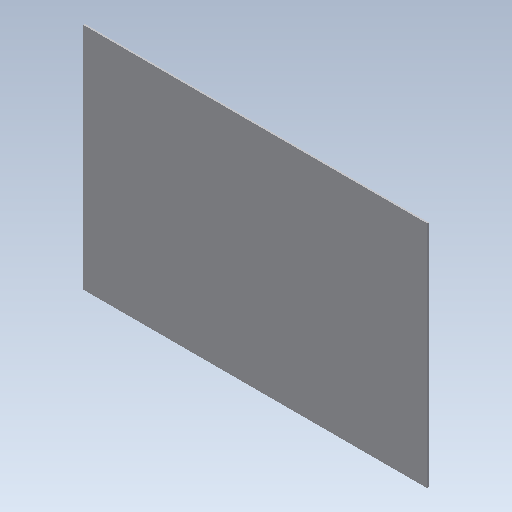
# Autodesk Inventor part: solar1
Saved by Autodesk Inventor 2020 (Build 240168000, 168)
## iProperties
Created: 2016-11-10
Part Number: solar1
Material: Aluminum 6061-AHC
Document SubType Name: Modeling
Designer: jous
Density: 2.71 g/cm^3
Appearance: Aluminum - Dark
Mass: 612.494 g
Surface Area: 2382.82 cm^2
Volume: 226.012 cm^3
Author: jous
Autodesk Inventor part; units mm, degrees
ref_plane "YZ Plane" through (0, 0, 0) normal (1, 0, 0) x (0, 1, 0)
ref_plane "XZ Plane" through (0, 0, 0) normal (0, 1, 0) x (-1, 0, 0)
ref_plane "XY Plane" through (0, 0, 0) normal (0, 0, 1) x (1, 0, 0)
sketch "Sketch1" plane through (0, 0, 0) normal (0, 0, 1) x (1, 0, 0)
  line L0 (-300, -140) -> (120, -140)
  line L1 (120, -140) -> (120, 140)
  line L2 (120, 140) -> (-300, 140)
  line L3 (-300, 140) -> (-300, -140)
  point P0 (0, 0)
  dimension "d0" = 420
  dimension "d1" = 280
  dimension "d36" = 300
  constraints: 8 end point, 2 parallel, 1 horizontal, 1 perpendicular
  measures "d0" distance of L2.end L1.end
  measures "d1" distance of L1.end L0.end
  measures "d36" distance from line of point (0, 0) L3
sketch "Sketch4" plane through (0, 0, 0) normal (0, 0, 1) x (1, 0, 0)
  line L0 (-273, -1) -> (-260.5, -1)
  line L1 (-148, -1) -> (-148, -13.5)
  line L2 (-148, -126) -> (-160.5, -126)
  line L3 (-273, -126) -> (-273, -113.5)
  line L4 (-273, -13.5) -> (-260.5, -1)
  line L5 (-160.5, -1) -> (-148, -13.5)
  line L6 (-148, -113.5) -> (-160.5, -126)
  line L7 (-260.5, -126) -> (-273, -113.5)
  line L8 (-260.5, -1) -> (-160.5, -1)
  line L9 (-273, -13.5) -> (-273, -1)
  line L10 (-160.5, -1) -> (-148, -1)
  line L11 (-148, -13.5) -> (-148, -113.5)
  line L12 (-160.5, -126) -> (-260.5, -126)
  line L13 (-148, -113.5) -> (-148, -126)
  line L14 (-260.5, -126) -> (-273, -126)
  line L15 (-273, -113.5) -> (-273, -13.5)
  line L16 (-300, -140) -> (120, -140) projected
  line L17 (-300, 140) -> (-300, -140) projected
  point P0 (0, 0)
  dimension "d6" = 125
  dimension "d7" = 125
  dimension "d8" = 12.5
  dimension "d9" = 12.5
  dimension "d10" = 12.5
  dimension "d11" = 12.5
  dimension "d12" = 12.5
  dimension "d13" = 12.5
  dimension "d14" = 12.5
  dimension "d15" = 12.5
  dimension "d22" = 14
  dimension "d23" = 27
  constraints: 32 end point, 18 parallel, 9 perpendicular, 3 horizontal, 3 point on line
  measures "d6" distance of L2.start L3.start
  measures "d7" distance of L1.start L2.start
  measures "d8" distance of L0.end L0.start
  measures "d9" distance of L1.start L5.start
  measures "d10" distance of L1.end L1.start
  measures "d11" distance of L2.start L6.start
  measures "d12" distance of L2.end L2.start
  measures "d13" distance of L3.start L7.start
  measures "d14" distance of L3.end L3.start
  measures "d15" distance of L4.start L0.start
  measures "d22" distance between parallel lines of L12 L16
  measures "d23" distance between parallel lines of L15 L17
sketch "Sketch5" plane through (0, 0, 0) normal (0, 0, 1) x (1, 0, 0)
  line L0 (-273, -13.5) -> (-260.5, -1) projected
  line L1 (-260.5, -1) -> (-160.5, -1) projected
  line L2 (-160.5, -1) -> (-148, -13.5) projected
  line L3 (-148, -13.5) -> (-148, -113.5) projected
  line L4 (-160.5, -126) -> (-260.5, -126) projected
  line L5 (-148, -113.5) -> (-160.5, -126) projected
  line L6 (-260.5, -126) -> (-273, -113.5) projected
  line L7 (-273, -113.5) -> (-273, -13.5) projected
  point P0 (0, 0)
boundary_patch "Boundary Patch3"
pattern_linear "Rectangular Pattern1" count 3 spacing 127 along (1, 0, 0) count 2 spacing 127 along (0, 1, 0) of "Boundary Patch3"
sketch "Sketch6" plane through (0, 0, 0) normal (0, 0, 1) x (1, 0, 0)
  line L0 (120, 140) -> (-300, 140) projected
  line L1 (-300, 140) -> (-300, -140) projected
  line L2 (-300, -140) -> (120, -140) projected
  line L3 (120, -140) -> (120, 140) projected
  line L4 (-260.5, 126) -> (-160.5, 126) projected
  line L5 (-133.5, 126) -> (-33.5, 126) projected
  line L6 (-146, 113.5) -> (-133.5, 126) projected
  line L7 (-160.5, 126) -> (-148, 113.5) projected
  line L8 (-273, 13.5) -> (-273, 113.5) projected
  line L9 (-273, 113.5) -> (-260.5, 126) projected
  line L10 (-260.5, 1) -> (-273, 13.5) projected
  line L11 (-160.5, 1) -> (-260.5, 1) projected
  line L12 (-148, 113.5) -> (-148, 13.5) projected
  line L13 (-148, 13.5) -> (-160.5, 1) projected
  line L14 (-133.5, 1) -> (-146, 13.5) projected
  line L15 (-146, 13.5) -> (-146, 113.5) projected
  line L16 (-21, 113.5) -> (-21, 13.5) projected
  line L17 (-19, 13.5) -> (-19, 113.5) projected
  line L18 (-33.5, 126) -> (-21, 113.5) projected
  line L19 (-19, 113.5) -> (-6.5, 126) projected
  line L20 (-6.5, 126) -> (93.5, 126) projected
  line L21 (93.5, 126) -> (106, 113.5) projected
  line L22 (106, 113.5) -> (106, 13.5) projected
  line L23 (-273, -113.5) -> (-273, -13.5) projected
  line L24 (-273, -13.5) -> (-260.5, -1) projected
  line L25 (-160.5, -1) -> (-148, -13.5) projected
  line L26 (-260.5, -1) -> (-160.5, -1) projected
  line L27 (-146, -13.5) -> (-133.5, -1) projected
  line L28 (-33.5, -1) -> (-21, -13.5) projected
  line L29 (-133.5, -1) -> (-33.5, -1) projected
  line L30 (-33.5, 1) -> (-133.5, 1) projected
  line L31 (-21, 13.5) -> (-33.5, 1) projected
  line L32 (106, 13.5) -> (93.5, 1) projected
  line L33 (-6.5, 1) -> (-19, 13.5) projected
  line L34 (93.5, 1) -> (-6.5, 1) projected
  line L35 (-6.5, -1) -> (93.5, -1) projected
  line L36 (-19, -13.5) -> (-6.5, -1) projected
  line L37 (93.5, -1) -> (106, -13.5) projected
  line L38 (-160.5, -126) -> (-260.5, -126) projected
  line L39 (-148, -13.5) -> (-148, -113.5) projected
  line L40 (-146, -113.5) -> (-146, -13.5) projected
  line L41 (-21, -13.5) -> (-21, -113.5) projected
  line L42 (-19, -113.5) -> (-19, -13.5) projected
  line L43 (106, -13.5) -> (106, -113.5) projected
  line L44 (106, -113.5) -> (93.5, -126) projected
  line L45 (93.5, -126) -> (-6.5, -126) projected
  line L46 (-6.5, -126) -> (-19, -113.5) projected
  line L47 (-21, -113.5) -> (-33.5, -126) projected
  line L48 (-33.5, -126) -> (-133.5, -126) projected
  line L49 (-133.5, -126) -> (-146, -113.5) projected
  line L50 (-148, -113.5) -> (-160.5, -126) projected
  line L51 (-260.5, -126) -> (-273, -113.5) projected
  point P0 (0, 0)
sketch "Sketch9" plane through (0, 0, 0) normal (0, 0, 1) x (1, 0, 0)
  line L0 (-260.5, 126) -> (-160.5, 126) projected
  line L1 (-160.5, 126) -> (-148, 113.5) projected
  line L2 (-148, 113.5) -> (-148, 13.5) projected
  line L3 (-273, 13.5) -> (-273, 113.5) projected
  line L4 (-273, 113.5) -> (-260.5, 126) projected
  line L5 (-160.5, 1) -> (-260.5, 1) projected
  line L6 (-260.5, 1) -> (-273, 13.5) projected
  line L7 (-273, -13.5) -> (-260.5, -1) projected
  line L8 (-260.5, -1) -> (-160.5, -1) projected
  line L9 (-273, -113.5) -> (-273, -13.5) projected
  line L10 (-160.5, -1) -> (-148, -13.5) projected
  line L11 (-148, -13.5) -> (-148, -113.5) projected
  line L12 (-148, 13.5) -> (-160.5, 1) projected
  line L13 (-133.5, 1) -> (-146, 13.5) projected
  line L14 (-146, -13.5) -> (-133.5, -1) projected
  line L15 (-146, -113.5) -> (-146, -13.5) projected
  line L16 (-146, 13.5) -> (-146, 113.5) projected
  line L17 (-133.5, 126) -> (-33.5, 126) projected
  line L18 (-146, 113.5) -> (-133.5, 126) projected
  line L19 (-33.5, 126) -> (-21, 113.5) projected
  line L20 (-21, 113.5) -> (-21, 13.5) projected
  line L21 (-21, 13.5) -> (-33.5, 1) projected
  line L22 (-33.5, 1) -> (-133.5, 1) projected
  line L23 (-133.5, -1) -> (-33.5, -1) projected
  line L24 (-33.5, -126) -> (-133.5, -126) projected
  line L25 (-160.5, -126) -> (-260.5, -126) projected
  line L26 (-260.5, -126) -> (-273, -113.5) projected
  line L27 (-148, -113.5) -> (-160.5, -126) projected
  line L28 (-21, -113.5) -> (-33.5, -126) projected
  line L29 (-133.5, -126) -> (-146, -113.5) projected
  line L30 (-33.5, -1) -> (-21, -13.5) projected
  line L31 (-6.5, 1) -> (-19, 13.5) projected
  line L32 (106, 13.5) -> (93.5, 1) projected
  line L33 (93.5, -1) -> (106, -13.5) projected
  line L34 (106, 113.5) -> (106, 13.5) projected
  line L35 (93.5, 1) -> (-6.5, 1) projected
  line L36 (-6.5, -1) -> (93.5, -1) projected
  line L37 (93.5, -126) -> (-6.5, -126) projected
  line L38 (-19, -113.5) -> (-19, -13.5) projected
  line L39 (-21, -13.5) -> (-21, -113.5) projected
  line L40 (106, -13.5) -> (106, -113.5) projected
  line L41 (-19, -13.5) -> (-6.5, -1) projected
  line L42 (-19, 13.5) -> (-19, 113.5) projected
  line L43 (-6.5, 126) -> (93.5, 126) projected
  line L44 (-19, 113.5) -> (-6.5, 126) projected
  line L45 (93.5, 126) -> (106, 113.5) projected
  line L46 (106, -113.5) -> (93.5, -126) projected
  line L47 (-6.5, -126) -> (-19, -113.5) projected
extrude "Extrusion4" add sketch "Sketch6" against normal blind 2
extrude "Extrusion6" add sketch "Sketch9" against normal blind 1.9
equation "\"d9\" = d8"
equation "\"d10\" = d9"
equation "\"d11\" = d10"
equation "\"d12\" = d11"
equation "\"d13\" = d12"
equation "\"d14\" = d13"
equation "\"d15\" = d8"
body "Solid4"
body "Srf3"
body "Srf4"
body "Srf5"
body "Srf8"
body "Srf9"
body "Srf10"
